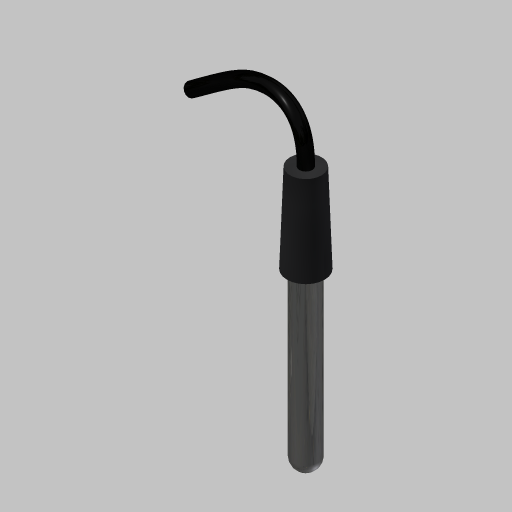
# Autodesk Inventor part: TempSensor_RS-762-1134
Saved by Autodesk Inventor 2023 (Build 270158000, 158)
## iProperties
Created: 2018-03-16
Part Number: TempSensor_RS-762-1134
Material: Generisch
Document SubType Name: Modeling
Designer: splath
Density: 1 g/cm^3
Appearance: Vorgabe
Author: splath
Autodesk Inventor part; units mm, degrees
note: some values were not read from the file. Chosen so that the rebuilt part matches the saved one: second side of "Extrusion1".
ref_plane "YZ Plane" through (0, 0, 0) normal (1, 0, 0) x (0, 1, 0)
ref_plane "XZ Plane" through (0, 0, 0) normal (0, 1, 0) x (-1, 0, 0)
ref_plane "XY Plane" through (0, 0, 0) normal (0, 0, 1) x (1, 0, 0)
sketch "Sketch1" plane through (0, 0, 0) normal (0, 0, 1) x (1, 0, 0)
  circle A0 centre (0, 0) radius 1.5
  dimension "d0" = 3
  constraints: 1 centre point, 1 coincident
  measures "d0" diameter of A0
extrude "Extrusion1" add sketch "Sketch1" against normal blind 30.8
fillet "Fillet1" radius 1.5 1 edges at (-1.5, 0, -30.8)
sketch "Sketch2" plane through (0, 0, 0) normal (0, 0, 1) x (1, 0, 0)
  circle A0 centre (0, 0) radius 0.7641
  constraints: 1 centre point, 1 coincident
sketch "Sketch3" plane through (0, 0, 0) normal (0, 1, 0) x (-1, 0, 0)
  line L0 (0, 0) -> (0, 4.4513) construction
  line L1 (0, 4.4513) -> (3.2656, 6.9674) construction
  line L2 (3.2656, 6.9674) -> (6.7058, 6) construction
  line L3 (6.7058, 6) -> (9.3195, 4.0867) construction
  line L4 (9.3195, 4.0867) -> (13.4254, 1.081) construction
  spline S0 degree 4 poles (0, 0) (0, 4.4513) (3.2656, 6.9674) (6.7058, 6) (9.3195, 4.0867) (13.4254, 1.081) knots 1 1 1 1 1 2 3 3 3 3 3
  line L5 (-1.5, 0) -> (1.5, 0) projected
  dimension "d11" = 6
  constraints: 1 point on line, 1 vertical, 3 other
  measures "d11" distance from line of L2.end L5
sweep "Sweep1" add profiles "Sketch2" path "Sketch3" path curves S0
sketch "Sketch4" plane through (0, 0, 0) normal (0, 0, 1) x (1, 0, 0)
  circle A0 centre (0, 0) radius 1.85
  circle A1 centre (0, 0) radius 1.5 projected
  dimension "d8" = 3.7
  constraints: 1 centre point, 1 coincident
  measures "d8" diameter of A0
extrude "Extrusion2" add sketch "Sketch4" against normal blind 10.4 draft 2 contours A0 | A1
body "Solid1"
